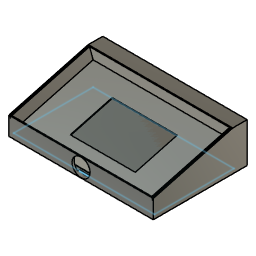
Sketch 2.1 v3 (Autodesk Fusion 360 design; units mm, degrees)
Autodesk Fusion 360 part; units mm, degrees
sketch "Sketch1" plane through (0, 0, 0) normal (0, 0, 1) x (1, 0, 0)
  line L0 (55.2242, 100.1802) -> (-54.7758, 100.1802)
  line L1 (-54.7758, 100.1802) -> (-54.7758, -99.8198)
  line L2 (-54.7758, -99.8198) -> (55.2242, -99.8198)
  line L3 (55.2242, -99.8198) -> (55.2242, 100.1802)
  dimension "d1" = 110
  dimension "d2" = 200
  constraint horizontal L0
  constraint vertical L1
  constraint horizontal L2
  constraint vertical L3
  measures "d1" distance of L0.start L0.end
  measures "d2" distance of L0.start L2.end
extrude "Extrude1" add sketch "Sketch1" along normal blind 55 makes body 1
move_body "Move1" bodies 1 to x (0, -1, 0) y (1, 0, 0) z (0, 0, 1) at (45.0439, -154.5956, 0)
move_body "Move2" bodies 1 to x (1, 0, 0) y (0, 1, 0) z (0, 0, 1) at (-45, 160, 0)
move_body "Move3" bodies 1 to x (1, 0, 0) y (0, 1, 0) z (0, 0, 1) at (0, -5, 0)
extrude "Extrude2" add 1 faces at (33.5575, 55.1802, 36.6667) along direction (0, 1, 0) blind 20 on bodies 1 bodies 1
chamfer "Chamfer1" distance 110 angle 15 1 edges at (0.2242, -54.8198, 55) measured on face at (33.5575, 31.8469, 55) on bodies 1
shell "Shell2" thickness 3 removed faces 0 bodies 1
sketch "Sketch2" plane through (0, -10.0536, 37.5206) normal (0, -0.258819, 0.965926) x (1, 0, 0)
  line L0 (100.2242, -46.3453) -> (100.2242, 67.5351)
  line L1 (100.2242, 67.5351) -> (-99.7758, 67.5351)
  line L2 (-99.7758, 67.5351) -> (-99.7758, -46.3453)
  line L3 (-99.7758, -46.3453) -> (100.2242, -46.3453)
  line L4 (-94.8529, 63.0754) -> (95.1471, 63.0754)
  line L5 (95.1471, 63.0754) -> (95.1471, -41.9246)
  line L6 (95.1471, -41.9246) -> (-94.8529, -41.9246)
  line L7 (-94.8529, -41.9246) -> (-94.8529, 63.0754)
  dimension "d11" = 190
  dimension "d12" = 105
  constraint horizontal L4
  constraint vertical L5
  constraint horizontal L6
  constraint vertical L7
  measures "d11" distance of L4.start L4.end
  measures "d12" distance of L4.start L6.end
extrude "Extrude3" cut sketch "Sketch2" against normal blind 10 contours L4 L5 L6 L7 bodies 1
extrude "Extrude4" cut 1 faces at (98.5318, 17.0777, 44.7904) along direction (0, 0.258819, -0.965926) blind 20 on bodies 1 bodies 1
sketch "Sketch3" plane through (0, -4.8772, 18.2021) normal (0, -0.258819, 0.965926) x (1, 0, 0)
  line L0 (-96.7758, -46.3453) -> (-96.7758, 67.5351)
  line L1 (-96.7758, 67.5351) -> (-99.7758, 67.5351)
  line L2 (-99.7758, 67.5351) -> (-99.7758, -46.3453)
  line L3 (-99.7758, -46.3453) -> (-96.7758, -46.3453)
  line L4 (-99.7758, 67.5351) -> (-98.2758, 67.5351)
  line L5 (-98.2758, 67.5351) -> (-98.2758, -46.3453)
  line L6 (-98.2758, -46.3453) -> (-99.7758, -46.3453)
  line L7 (-99.7758, -46.3453) -> (-99.7758, 67.5351)
  constraint horizontal L4
  constraint vertical L5
  constraint horizontal L6
  constraint vertical L7
  constraint midpoint L3 L5.end
  constraint coincident L1.end L2.start
extrude "Extrude5" add sketch "Sketch3" along normal blind 20 contours L1 L2 L3 L4 L5 L6 L7 bodies 1
sketch "Sketch4" plane through (0, -4.8772, 18.2021) normal (0, -0.258819, 0.965926) x (1, 0, 0)
  line L0 (97.2242, 67.5351) -> (97.2242, -46.3453)
  line L1 (97.2242, -46.3453) -> (100.2242, -46.3453)
  line L2 (100.2242, -46.3453) -> (100.2242, 67.5351)
  line L3 (100.2242, 67.5351) -> (97.2242, 67.5351)
  line L4 (100.2242, 67.5351) -> (98.7242, 67.5351)
  line L5 (98.7242, 67.5351) -> (98.7242, -46.3453)
  line L6 (98.7242, -46.3453) -> (100.2242, -46.3453)
  line L7 (100.2242, -46.3453) -> (100.2242, 67.5351)
  dimension "d19" = 1.5
  constraint horizontal L4
  constraint vertical L5
  constraint horizontal L6
  constraint vertical L7
  constraint coincident L2.end L3.start
  measures "d19" distance of L2.end L4.end
extrude "Extrude6" add sketch "Sketch4" along normal blind 20 contours L1 L2 L3 L4 L5 L6 L7 bodies 1
sketch "Sketch5" plane through (0, 0, 3) normal (0, 0, 1) x (-1, 0, 0)
  line L0 (96.7758, 51.8198) -> (-97.2242, 51.8198)
  line L1 (-97.2242, 51.8198) -> (-97.2242, -72.1802)
  line L2 (-97.2242, -72.1802) -> (96.7758, -72.1802)
  line L3 (96.7758, -72.1802) -> (96.7758, 51.8198)
sketch "Sketch1 (2)" plane through (0, 0, 3) normal (0, 0, 1) x (1, 0, 0) in component "Screen holder"
  line L0 (97.6714, 59.4316) -> (-97.3286, 59.4316)
  line L1 (-97.3286, 59.4316) -> (-97.3286, -50.5684)
  line L2 (-97.3286, -50.5684) -> (97.6714, -50.5684)
  line L3 (97.6714, -50.5684) -> (97.6714, 59.4316)
  dimension "d22" = 195
  dimension "d23" = 110
  constraint horizontal L0
  constraint vertical L1
  constraint horizontal L2
  constraint vertical L3
  measures "d22" distance of L0.start L0.end
  measures "d23" distance of L0.start L2.end
extrude "Extrude1'" add sketch "Sketch5" along normal blind 20 separate body makes body 2 in component "Screen holder"
extrude "Extrude2'" cut 1 faces at (32.5575, 72.1802, 9.6667) along direction (0, -1, 0) blind 11.5 on bodies 2 bodies 2 in component "Screen holder"
move_body "Move1'" bodies 2 to x (1, 0, 0) y (0, 0.965926, 0.258819) z (0, -0.258819, 0.965926) at (0, 8.4112, 17.0683) in component "Screen holder"
move_body "Move2'" bodies 2 to x (1, 0, 0) y (0, 1, 0) z (0, 0, 1) at (0, -6, -0.25) in component "Screen holder"
extrude "Extrude3'" add 1 faces at (97.2242, -13.9226, 22.4493) along direction (1, 0, 0) blind 2 on bodies 2 bodies 2 in component "Screen holder"
move_body "Move3'" bodies 2 to x (1, 0, 0) y (0, 1, 0) z (0, 0, 1) at (-1, 0, 0) in component "Screen holder"
extrude "Extrude4'" add 1 faces at (-32.4425, -50.1448, 12.7436) along direction (0, -0.965926, -0.258819) blind 1 on bodies 2 bodies 2 in component "Screen holder"
move_body "Move4" bodies 2 to x (1, 0, 0) y (0, 1, 0) z (0, 0, 1) at (0, -0.2, 0.3) in component "Screen holder"
shell "Shell1" thickness 1 removed faces 1 at (-32.4425, -18.2174, 35.4558) on bodies 2 in component "Screen holder"
sketch "Sketch2 (2)" plane through (0, -5.1667, 19.2825) normal (0, -0.258819, 0.965926) x (1, 0, 0) in component "Screen holder"
  line L0 (97.2242, 66.2466) -> (-96.7758, 66.2466)
  line L1 (-96.7758, 66.2466) -> (-96.7758, -45.2534)
  line L2 (-96.7758, -45.2534) -> (97.2242, -45.2534)
  line L3 (97.2242, -45.2534) -> (97.2242, 66.2466)
  line L4 (-45, 40) -> (45, 40)
  line L5 (45, 40) -> (45, -20)
  line L6 (45, -20) -> (-45, -20)
  line L7 (-45, -20) -> (-45, 40)
  dimension "d33" = 90
  dimension "d34" = 60
  constraint horizontal L4
  constraint vertical L5
  constraint horizontal L6
  constraint vertical L7
  measures "d33" distance of L4.start L4.end
  measures "d34" distance of L4.start L6.end
extrude "Extrude5'" cut sketch "Sketch2 (2)" against normal blind 15 contours L4 L5 L6 L7 bodies 2 in component "Screen holder"
hole "Hole1" at (0.2242, -54.8198, 12.7628) direction (0, 1, 0) diameter 25 depth 6 tip angle 180 bodies 1
hole "Hole1'" [no effect] in component "Screen holder"
hole "Hole2" at (-99.7758, -48.171, 9.8923) direction (1, 0, 0) diameter 0.318 depth 9 tip angle 180 countersink diameter 2 countersink angle 90 bodies 1
thread "Thread1" "ISO Metric profile 0.4 M0.4x0.1 6H"
thread "Thread1'" "ISO Metric profile 0.4 M0.4x0.1 6H" in component "Screen holder"
hole "Hole2'" at (-99.7758, -48.171, 9.8923) direction (1, 0, 0) diameter 0.318 depth 9 tip angle 180 countersink diameter 2 countersink angle 90 bodies 2 in component "Screen holder"
sketch "Sketch3 (2)" plane through (0, 75.1802, 0) normal (0, 1, 0) x (-1, 0, 0) in component "Screen holder"
  line L0 (-100.2242, 0) -> (99.7758, 0)
  line L1 (99.7758, 0) -> (99.7758, 55)
  line L2 (99.7758, 55) -> (-100.2242, 55)
  line L3 (-100.2242, 55) -> (-100.2242, 0)
  line L4 (45, 30) -> (44, 30)
  line L5 (44, 30) -> (44, 5)
  line L6 (44, 5) -> (45, 5)
  line L7 (45, 5) -> (45, 30)
  dimension "d55" = 1
  dimension "d56" = 25
  dimension "d57" = 54.7758
  dimension "d58" = 5
  constraint horizontal L4
  constraint vertical L5
  constraint horizontal L6
  constraint vertical L7
  measures "d55" distance of L4.start L4.end
  measures "d56" distance of L4.start L6.end
  measures "d57" distance of L1 L7
  measures "d58" distance of L0 L6
extrude "Extrude7" cut sketch "Sketch3 (2)" against normal blind 3 contours L4 L5 L6 L7 bodies 1
pattern_linear "R-Pattern1" count 1 spacing 0 along (0, 0, -1) count 30 spacing 3.069 along (1, 0, 0) of "Extrude7"
component "Screen holder" placed x (1, 0, 0) y (0, 1, 0) z (0, 0, 1) at (0, 0, 0)
